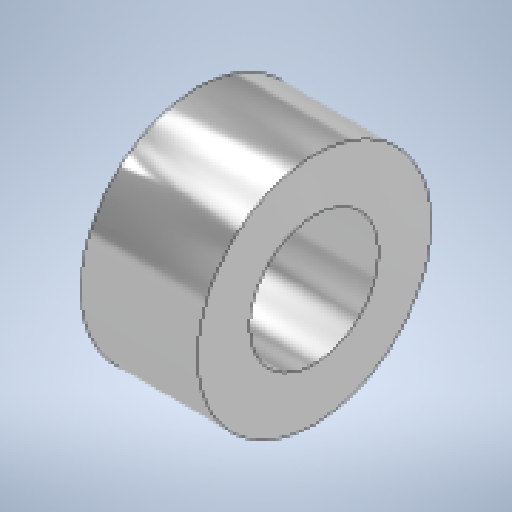
# Autodesk Inventor part: Lever
Saved by Autodesk Inventor 2023.2 (Build 272271000, 271)
## iProperties
Created: 2024-03-17
Part Number: Lever
Material: Aluminum 6061
Document SubType Name: Modeling
Designer: Nathan Cai
Mass: 1.01002 g
Surface Area: 5.27592 cm^2
Volume: 0.374081 cm^3
Density: 2.7 g/cm^3
Appearance: Aluminum - Flat
Author: Nathan Cai
Autodesk Inventor part; units mm, degrees
ref_plane "YZ Plane" through (0, 0, 0) normal (1, 0, 0) x (0, 1, 0)
ref_plane "XZ Plane" through (0, 0, 0) normal (0, 1, 0) x (-1, 0, 0)
ref_plane "XY Plane" through (0, 0, 0) normal (0, 0, 1) x (1, 0, 0)
sketch "Sketch1" plane through (0, 0, 0) normal (1, 0, 0) x (0, 1, 0)
  circle A0 centre (0, 0) radius 1.7526
  circle A1 centre (0, 0) radius 3.175
  circle A2 centre (2.0674, 6.004) radius 3.5 construction
  circle A3 centre (2.0674, 6.004) radius 1.5
  circle A4 centre (2.0674, 6.004) radius 2.5
  line L0 (-2.8751, 1.3469) -> (-0.1965, 7.0646)
  line L1 (0, 0) -> (15.875, 1.6685) construction
  line L2 (0, 0) -> (3.175, 0) construction
  line L3 (3.0949, -0.7087) -> (4.5043, 5.446)
  circle A5 centre (16.0409, 0.0897) radius 1.5875
  line L4 (15.875, 1.6685) -> (3.3375, 0.3508)
  line L5 (16.2069, -1.4891) -> (0.3319, -3.1576)
  line L6 (2.0674, 6.004) -> (0, 0) construction
  line L7 (2.0674, 6.004) -> (3.4856, 5.5157) construction
  line L8 (0, 0) -> (1.6571, -0.5706) construction
  dimension "d0" = 3.5052
  dimension "d7" = 3
  dimension "d1" = 6.35
  dimension "d4" = 7
  dimension "d8" = 5
  dimension "d9" = 6
  dimension "d10" = 15.875
  dimension "d11" = 3.175
  dimension "d15" = 6.35
  dimension "d16" = 65
  constraints: 18 end point, 8 point on circle, 7 tangent, 4 centre point, 4 coincident, 2 perpendicular, 2 point on line, 1 horizontal, 6 other
  measures "d1" diameter of A1
  measures "d4" diameter of A2
  measures "d8" diameter of A4
  measures "d9" angle of L2 L1
  measures "d10" horizontal distance of L1.start L1.end
  measures "d11" diameter of A5
  measures "d15" distance between parallel lines of L7 L8
  measures "d16" angle of L6 L1
extrude "Extrusion1" add sketch "Sketch1" along normal blind 3.175
fillet "Fillet1" radius 6.35 1 edges at (1.5875, 3.3375, 0.3508)
sketch "Sketch2" plane through (0, 0, 0) normal (-1, 0, 0) x (0, 0, 1)
  circle A0 centre (6.004, 2.0674) radius 1.5 projected
  arc A1 (7.0646, -0.1965) -> (6.4319, 4.5305) centre (6.004, 2.0674) ccw projected
  circle A2 centre (6.004, 2.0674) radius 2.5
  point P0 (0, 0)
  point P1 (7.0646, -0.1965)
  constraints: 1 coincident, 3 other
extrude "Extrusion2" add sketch "Sketch2" along normal blind 3.175
body "Solid1"
